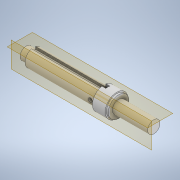
# Autodesk Inventor part: eixo beto terminado
Saved by Autodesk Inventor 2022.1 (Build 261234020, 234B)
## iProperties
Created: 2023-09-01
Part Number: eixo beto terminado
Material: Generic
Document SubType Name: Modeling
Designer: SENAI
Density: 1 g/cm^3
Appearance: Default
Author: SENAI
Autodesk Inventor part; units mm, degrees
ref_plane "YZ Plane" through (0, 0, 0) normal (1, 0, 0) x (0, 1, 0)
sketch "Sketch1" plane through (0, 0, 0) normal (0, 0, 1) x (1, 0, 0)
  line L0 (0, 0) -> (310, 0)
  line L1 (0, 0) -> (0, 12.5)
  line L2 (0, 12.5) -> (15, 12.5)
  line L3 (15, 12.5) -> (15, 17.5)
  line L4 (15, 17.5) -> (157, 17.5)
  line L5 (157, 17.5) -> (157, 23.1)
  line L6 (157, 23.1) -> (183, 23.1)
  line L7 (183, 23.1) -> (183, 20.8)
  line L8 (183, 20.8) -> (187, 20.8)
  line L9 (187, 20.8) -> (187, 12.8)
  line L10 (187, 12.8) -> (257.9994, 12.5)
  line L11 (257.9994, 12.5) -> (257.9994, 0)
  dimension "d0" = 310
  dimension "d1" = 12.5
  dimension "d2" = 15
  dimension "d3" = 5
  dimension "d4" = 142
  dimension "d5" = 5.6
  dimension "d6" = 26
  dimension "d7" = 2.3
  dimension "d8" = 4
  dimension "d9" = 8
  dimension "d10" = 71
  constraints: 24 end point, 8 perpendicular, 2 horizontal, 2 point on line, 1 vertical
  measures "d0" distance of L0.start L0.end
  measures "d1" distance of L0.start L1.end
  measures "d2" distance of L1.end L2.end
  measures "d3" distance of L2.end L3.end
  measures "d4" distance of L3.end L4.end
  measures "d5" distance of L4.end L5.end
  measures "d6" distance of L5.end L6.end
  measures "d7" distance of L6.end L7.end
  measures "d8" distance of L7.end L8.end
  measures "d9" distance of L8.end L9.end
  measures "d10" distance of L9.end L10.end
revolve "Revolution1" add sketch "Sketch1" angle 360 about axis through (0, 0, 0) along (1, 0, 0)
ref_plane "Work Plane1" through (0, 17.25, 0) normal (0, 1, 0) x (-1, 0, 0)
sketch "Sketch2" plane through (0, 17.25, 0) normal (0, 1, 0) x (-1, 0, 0)
  line L0 (-15, 4) -> (-165, 4)
  line L1 (-165, 4) -> (-165, -4)
  line L2 (-165, -4) -> (-15, -4)
  line L3 (-15, -4) -> (-15, 4)
  line L4 (-15, 17.5) -> (-15, -17.5) projected
  point P0 (0, 0)
  dimension "d15" = 150
  dimension "d16" = 150
  constraints: 8 end point, 2 perpendicular, 1 collinear
  measures "d15" distance of L0.start L0.end
  measures "d16" distance of L1.end L2.end
extrude "Extrusion1" cut sketch "Sketch2" along normal blind 6.25 and the other way blind 5
fillet "Fillet1" radius 11 1 edges at (165, 12.25, 0)
ref_plane "Work Plane2" through (86, 0, 17.5) normal (0, 0, 1) x (1, 0, 0)
sketch "Sketch3" plane through (86, 0, 17.5) normal (0, 0, 1) x (1, 0, 0)
  circle A0 centre (61.0014, 0) radius 4
  line L0 (71, -23.1) -> (71, 22.751) projected
  point P0 (-86, 0)
  dimension "d22" = 8
  constraints: 1 centre point
  measures "d22" diameter of A0
extrude "Extrusion2" cut sketch "Sketch3" against normal blind 40
body "Solid1"
